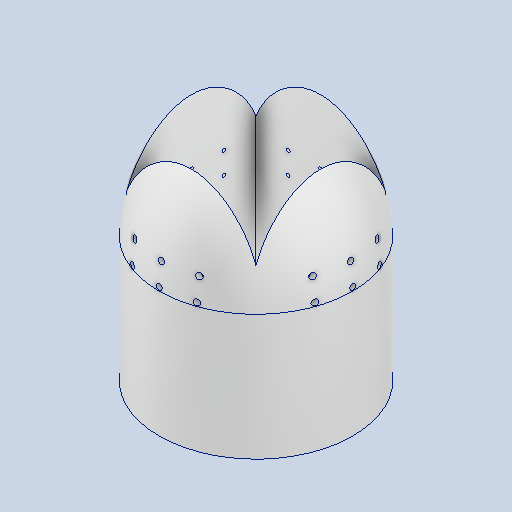
# Autodesk Inventor part: Model Shell_part2
Saved by Autodesk Inventor 2023 (Build 270158000, 158)
## iProperties
Created: 2023-03-19
Part Number: Model Shell_part2
Material: Aluminum 6061
Document SubType Name: Modeling
Designer: ASARe-DAQ-PC
Density: 2.7 g/cm^3
Appearance: Aluminum - Flat
Mass: 15017.9 g
Surface Area: 4822.32 cm^2
Volume: 5562.2 cm^3
Author: ASARe-DAQ-PC
Autodesk Inventor part; units mm, degrees
ref_plane "YZ Plane" through (0, 0, 0) normal (1, 0, 0) x (0, 1, 0)
ref_plane "XZ Plane" through (0, 0, 0) normal (0, 1, 0) x (-1, 0, 0)
ref_plane "XY Plane" through (0, 0, 0) normal (0, 0, 1) x (1, 0, 0)
sketch "Sketch2" plane through (0, 0, 0) normal (1, 0, 0) x (0, 1, 0)
  line L0 (0, 135) -> (175, 135)
  arc A0 (300, 90) -> (175, 135) centre (175, -61.1111) ccw
  line L1 (0, 135) -> (0, 0)
  line L2 (300, 90) -> (300, 0)
  line L3 (300, 0) -> (0, 0)
  line L4 (-60.7853, 0) -> (364.712, 0) projected
  point P0 (175, 130)
  dimension "d12" = 175
  dimension "d13" = 135
  dimension "d14" = 90
  dimension "d15" = 300
  constraints: 8 end point, 2 point on circle, 2 vertical, 1 centre point, 1 horizontal, 1 perpendicular, 1 tangent
  measures "d12" distance of L0.start L0.end
  measures "d13" distance from line of L1.end L0
  measures "d14" vertical distance of L1.end L2.start
  measures "d15" horizontal distance of L1.end L2.start
revolve "Revolution1" add sketch "Sketch2" angle 360 about axis through (0, -10, 0) along (0, 1, 0)
sketch "Sketch4" plane through (0, 0, 0) normal (0, -1, 0) x (1, 0, 0)
  circle A0 centre (0, 0) radius 130
  dimension "d21" = 260
  constraints: 1 centre point, 1 coincident
  measures "d21" diameter of A0
extrude "Extrusion2" cut sketch "Sketch4" against normal blind 30
sketch "Sketch5" plane through (0, 300, 0) normal (0, 1, 0) x (1, 0, 0)
  line L0 (90, -90) -> (-90, -90)
  line L1 (-90, -90) -> (-90, 90)
  line L2 (-90, 90) -> (90, 90)
  line L3 (90, 90) -> (90, -90)
  line L4 (90, -90) -> (-90, 90) construction
  line L5 (-90, -90) -> (90, 90) construction
  point P0 (0, 0)
  dimension "d24" = 180
  dimension "d25" = 180
  constraints: 12 end point, 2 midpoint, 2 parallel, 1 horizontal, 1 perpendicular
  measures "d24" distance of L0.start L0.end
  measures "d25" distance of L0.end L1.end
extrude "Extrusion3" cut sketch "Sketch5" against normal up to next
sketch "Sketch6" plane through (-90, 30, -90) normal (1, 0, 0) x (0, 0, -1)
  line L0 (40, -30) -> (-220, -30) projected
  line L1 (-180, 199.4853) -> (-180, 0) projected
  point P0 (-90, -30)
  point P1 (-135, 150)
  dimension "d35" = 180
  dimension "d36" = 45
  measures "d35" distance from line of point (-135, 150) L0
  measures "d36" distance from line of point (-135, 150) L1
hole "Hole1" at (-90, 180, 45) direction (-1, 0, 0) diameter 5 depth 28
pattern_linear "Rectangular Pattern1" count 3 spacing 45 along (0, 0, -1) of "Hole1"
ref_plane "Work Plane1" through (-90, 300, 90) normal (0.7071068, 0, 0.7071068) x (0, -1, 0)
mirror "Mirror1" about plane through (0, 0, 0) normal (1, 0, 0) of "Hole1", "Rectangular Pattern1"
mirror "Mirror2" about plane through (-90, 300, 90) normal (0.7071068, 0, 0.7071068) of "Hole1", "Rectangular Pattern1", "Mirror1"
sketch "Sketch10" plane through (-118, 180, 0) normal (1, 0, 0) x (0, 0, -1)
  circle A0 centre (0, 0) radius 2.5 projected
  point P0 (0, -180)
  constraints: 1 coincident
hole "Hole4" at (-118, 180, 0) direction (-1, 0, 0) diameter 8 end through all
pattern_linear "Rectangular Pattern2" count 2 spacing 45 along (0, 0, 1) count 2 spacing 45 along (0, 0, -1) of "Hole4"
mirror "Mirror3" about plane through (0, 0, 0) normal (1, 0, 0) of "Rectangular Pattern2"
mirror "Mirror4" about plane through (-90, 300, 90) normal (0.7071068, 0, 0.7071068) of "Rectangular Pattern2", "Mirror3"
pattern_linear "Rectangular Pattern3" count 2 spacing 30 along (0, 1, 0) of "Hole1", "Rectangular Pattern1", "Mirror1", "Mirror2", "Hole4", "Rectangular Pattern2", "Mirror3", "Mirror4"
body "Solid2"
